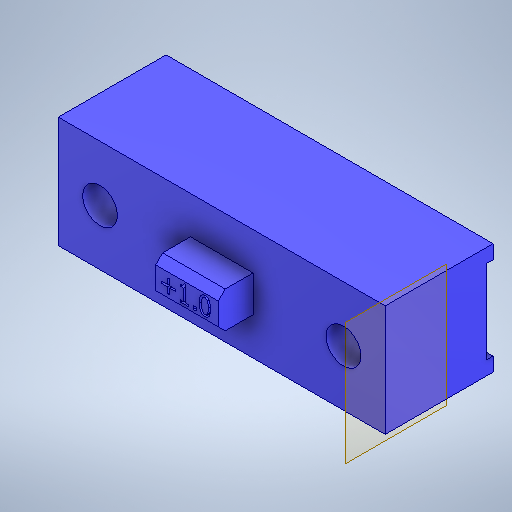
# Autodesk Inventor part: Bearing Spacer_V2_1mm
Saved by Autodesk Inventor 2025.4 (Build 294407000, 407)
## iProperties
Created: 2026-06-01
Part Number: Bearing Spacer_V2_1mm
Material: 일반
Document SubType Name: Modeling
Designer: dalbi
Density: 1 g/cm^3
Appearance: 기본값
Author: dalbi
Autodesk Inventor part; units mm, degrees
ref_plane "YZ Plane" through (0, 0, 0) normal (1, 0, 0) x (0, 1, 0)
ref_plane "XZ Plane" through (0, 0, 0) normal (0, 1, 0) x (-1, 0, 0)
ref_plane "XY Plane" through (0, 0, 0) normal (0, 0, 1) x (1, 0, 0)
ref_plane "작업 평면1" through (23.5, -8, -2) normal (1, 0, 0) x (0, 0, -1)
sketch "스케치1" plane through (23.5, -8, -2) normal (1, 0, 0) x (0, 0, -1)
  line L0 (0, 16) -> (-8.15, 16) projected
  line L1 (-8.15, 16) -> (-8.15, 10.6) projected
  line L2 (-8.15, 10.6) -> (-12.15, 10.6) projected
  line L3 (-13.15, 9.6) -> (-12.15, 10.6) projected
  line L4 (-13.15, 9.6) -> (-13.15, 6.4) projected
  line L5 (-12.15, 5.4) -> (-13.15, 6.4) projected
  line L6 (-12.15, 5.4) -> (-8.15, 5.4) projected
  line L7 (-8.15, 5.4) -> (-8.15, 0) projected
  line L8 (-8.15, 0) -> (0, 0) projected
  line L9 (0, 16) -> (7.35, 16)
  line L10 (7.35, 16) -> (7.35, 15)
  line L11 (0, 0) -> (7.35, 0)
  line L12 (7.35, 0) -> (7.35, 1)
  line L13 (0, 16) -> (-8.15, 16)
  line L14 (-8.15, 10.6) -> (-12.15, 10.6) projected
  line L15 (-8.15, 10.6) -> (-12.15, 10.6)
  line L16 (-12.15, 10.6) -> (-13.15, 9.6)
  line L17 (-13.15, 6.4) -> (-12.15, 5.4)
  line L18 (6.35, 14) -> (7.35, 14)
  line L19 (7.35, 14) -> (7.35, 15)
  line L20 (6.35, 2) -> (7.35, 2)
  line L21 (7.35, 2) -> (7.35, 1)
  line L22 (6.35, 14) -> (6.35, 2)
  point P0 (-2, 8)
  point P1 (4.35, 10.6)
  point P2 (4.35, 5.4)
  dimension "d1" = 7.35
  dimension "d13" = 7.35
  constraints: 26 end point, 5 perpendicular, 4 horizontal, 2 collinear, 2 point on line
  measures "d1" distance of L0.start L9.end
  measures "d13" distance of L8.end L11.end
sketch "스케치2" plane through (-23.5, 8, 6.15) normal (0, 0, 1) x (1, 0, 0)
  arc A0 (7.9209, -9.6) -> (7.9209, -6.4) centre (6, -8) ccw projected
  line L0 (39.0791, -9.6) -> (7.9209, -9.6) projected
  circle A1 centre (6, -8) radius 2.5
  circle A2 centre (41, -8) radius 2.5 projected
  circle A3 centre (41, -8) radius 2.5
  point P0 (23.5, -8)
  point P1 (7.9209, -6.4)
  constraints: 2 coincident, 1 centre point, 4 other
extrude "돌출1" add sketch "스케치1" against normal up to surface (47 mm away)
extrude "돌출2" cut sketch "스케치2" along normal mid plane 50
sketch "스케치3" plane through (-15.5791, 1.6, 11.15) normal (0, 0, 1) x (1, 0, 0)
  line L0 (15.5791, -14.4593) -> (15.5791, 15.5737)
  line L1 (-7.9209, 4.4) -> (-7.9209, -7.6) projected
  line L2 (-7.9209, 4.4) -> (11.0791, 4.4)
  line L3 (11.0791, 4.4) -> (11.0791, -7.6)
  line L4 (11.0791, -7.6) -> (-7.9209, -7.6)
  line L5 (-7.9209, -7.6) -> (-7.9209, 4.4)
  line L6 (39.0791, 4.4) -> (39.0791, -7.6)
  line L7 (39.0791, 4.4) -> (20.0791, 4.4)
  line L8 (20.0791, 4.4) -> (20.0791, -7.6)
  line L9 (20.0791, -7.6) -> (39.0791, -7.6)
  line L10 (39.0791, -7.6) -> (39.0791, 4.4)
  point P0 (15.5791, -1.6)
  dimension "d9" = 19
  constraints: 20 end point, 5 symmetric about line, 2 parallel, 1 horizontal, 1 perpendicular, 1 vertical
  measures "d9" distance of L1.start L2.end
extrude "돌출3" cut sketch "스케치3" against normal up to surface (5 mm away)
sketch "스케치4" plane through (-4.5, 1.6, 11.15) normal (0, 0, 1) x (1, 0, 0)
  line L0 (0.6181, -0.2528) -> (7.2489, -0.2528) construction
  line L1 (7.2489, -0.2528) -> (7.2489, -2.6222) construction
  line L2 (7.2489, -2.6222) -> (0.6181, -2.6222) construction
  line L3 (0.6181, -2.6222) -> (0.6181, -0.2528) construction
  line L4 (2.8925, -1.8686) -> (2.0321, -1.8686)
  line L5 (2.0321, -1.8686) -> (2.0321, -2.729)
  line L6 (2.0321, -2.729) -> (1.7481, -2.729)
  line L7 (1.7481, -2.729) -> (1.7481, -1.8686)
  line L8 (1.7481, -1.8686) -> (0.8877, -1.8686)
  line L9 (0.8877, -1.8686) -> (0.8877, -1.5949)
  line L10 (0.8877, -1.5949) -> (1.7481, -1.5949)
  line L11 (1.7481, -1.5949) -> (1.7481, -0.7345)
  line L12 (1.7481, -0.7345) -> (2.0321, -0.7345)
  line L13 (2.0321, -0.7345) -> (2.0321, -1.5949)
  line L14 (2.0321, -1.5949) -> (2.8925, -1.5949)
  line L15 (2.8925, -1.5949) -> (2.8925, -1.8686)
  line L16 (4.7842, -2.8443) -> (3.545, -2.8443)
  line L17 (3.545, -2.8443) -> (3.545, -2.5849)
  line L18 (3.545, -2.5849) -> (4.0061, -2.5849)
  line L19 (4.0061, -2.5849) -> (4.0061, -0.8827)
  line L20 (4.0061, -0.8827) -> (3.545, -0.8827)
  line L21 (3.545, -0.8827) -> (3.545, -0.6501)
  spline S0 degree 2 poles (3.545, -0.6501) (3.8064, -0.6501) (4.0534, -0.5019) (4.0699, -0.2961) knots 0 0 0 1 2 2 2
  line L22 (4.0699, -0.2961) -> (4.3334, -0.2961)
  line L23 (4.3334, -0.2961) -> (4.3334, -2.5849)
  line L24 (4.3334, -2.5849) -> (4.7842, -2.5849)
  line L25 (4.7842, -2.5849) -> (4.7842, -2.8443)
  line L26 (5.7969, -2.8443) -> (5.3893, -2.8443)
  line L27 (5.3893, -2.8443) -> (5.3893, -2.3585)
  line L28 (5.3893, -2.3585) -> (5.7969, -2.3585)
  line L29 (5.7969, -2.3585) -> (5.7969, -2.8443)
  spline S1 degree 2 poles (7.8902, -1.5743) (7.8902, -2.2577) (7.4929, -2.8978) (7.0792, -2.8978) knots 0 0 0 1 2 2 2
  spline S2 degree 2 poles (7.0792, -2.8978) (6.6593, -2.8978) (6.2662, -2.2453) (6.2662, -1.5763) knots 0 0 0 1 2 2 2
  spline S3 degree 2 poles (6.2662, -1.5763) (6.2662, -0.8889) (6.6634, -0.2528) (7.0792, -0.2528) knots 0 0 0 1 2 2 2
  spline S4 degree 2 poles (7.0792, -0.2528) (7.4971, -0.2528) (7.8902, -0.9115) (7.8902, -1.5743) knots 0 0 0 1 2 2 2
  spline S5 degree 2 poles (7.4538, -2.3482) (7.5032, -2.2227) (7.5444, -1.8357) (7.5444, -1.5743) knots 0 0 0 1 2 2 2
  spline S6 degree 2 poles (7.5444, -1.5743) (7.5444, -1.3129) (7.5032, -0.928) (7.4518, -0.7983) knots 0 0 0 1 2 2 2
  spline S7 degree 2 poles (7.4518, -0.7983) (7.4003, -0.6686) (7.2212, -0.5348) (7.0792, -0.5348) knots 0 0 0 1 2 2 2
  spline S8 degree 2 poles (7.0792, -0.5348) (6.9372, -0.5348) (6.754, -0.6686) (6.7005, -0.8024) knots 0 0 0 1 2 2 2
  spline S9 degree 2 poles (6.7005, -0.8024) (6.649, -0.9321) (6.612, -1.3273) (6.612, -1.5763) knots 0 0 0 1 2 2 2
  spline S10 degree 2 poles (6.612, -1.5763) (6.612, -1.8439) (6.6449, -2.2021) (6.6984, -2.342) knots 0 0 0 1 2 2 2
  spline S11 degree 2 poles (6.6984, -2.342) (6.7478, -2.4738) (6.931, -2.6158) (7.0792, -2.6158) knots 0 0 0 1 2 2 2
  spline S12 degree 2 poles (7.0792, -2.6158) (7.2192, -2.6158) (7.4024, -2.482) (7.4538, -2.3482) knots 0 0 0 1 2 2 2
  point P0 (4.5, -1.6)
  constraints: 2 other
extrude "돌출4" cut sketch "스케치4" against normal blind 5
